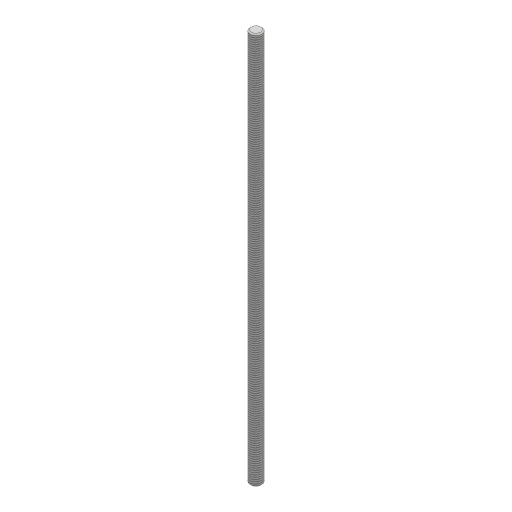
# Autodesk Inventor part: COTS_GENERIC_M6_Threaded_Rod_200mm
Saved by Autodesk Inventor 2024.3 (Build 283343000, 343)
## iProperties
Created: 2018-02-17
Part Number: COTS_GENERIC_M6_Threaded_Rod_200mm
Material: Ogólny
Document SubType Name: Modeling
Designer: Andrzej
Density: 1 g/cm^3
Appearance: Domyślna
Mass: 5.64853 g
Surface Area: 38.1227 cm^2
Volume: 5.64853 cm^3
Author: Andrzej
Autodesk Inventor part; units mm, degrees
ref_plane "YZ Plane" through (0, 0, 0) normal (1, 0, 0) x (0, 1, 0)
ref_plane "XZ Plane" through (0, 0, 0) normal (0, 1, 0) x (-1, 0, 0)
ref_plane "XY Plane" through (0, 0, 0) normal (0, 0, 1) x (1, 0, 0)
sketch "Szkic1" plane through (0, 0, 0) normal (0, 0, 1) x (1, 0, 0)
  circle A0 centre (0, 0) radius 3
  dimension "d0" = 6
  constraints: 1 centre point, 1 coincident
  measures "d0" diameter of A0
extrude "Wyciągnięcie proste1" add sketch "Szkic1" along normal blind 200
chamfer "Faza1" distance 0.6 angle 45 2 edges at (-3, 0, 0) (-3, 0, 200)
thread "Gwint1" size "M6x1" class "6g" standard "ANSI Metric M Profile" full length
